screw v2 (Autodesk Fusion 360 design; units mm, degrees)
Autodesk Fusion 360 part; units mm, degrees
note: some values were not read from the file. Set by a fixed rule: which sketch regions a step uses.
sketch "Sketch1" plane through (0, 0, 0) normal (0, 0, 1) x (1, 0, 0)
  circle A0 centre (0, 0) radius 5.574
  dimension "d2" = 11.148
  constraint coincident A0.centre origin
  measures "d2" diameter of A0
extrude "Extrude1" add sketch "Sketch1" along normal blind 15
thread "Thread1" "ISO Metric Trapezoidal Threads 14.0 TR14x3 7e" major diameter 13.882 minor diameter 10.3175 pitch 3 angle 30 modelled right hand crest width 1.0769 on face at (5.5463, -0.555, 10) crest through (6.941, 0, -0.75)
sketch "Sketch2" plane through (0, 0, 15) normal (0, 0, 1) x (-1, 0, 0)
  line L0 (-10, 0) -> (-5, -8.6603)
  line L1 (-5, -8.6603) -> (5, -8.6603)
  line L2 (5, -8.6603) -> (10, 0)
  line L3 (10, 0) -> (5, 8.6603)
  line L4 (5, 8.6603) -> (-5, 8.6603)
  line L5 (-5, 8.6603) -> (-10, 0)
  spline S0 degree 3 poles (6.2708, -2.9757) (6.4311, -2.1502) (6.4357, -1.3016) (6.1375, 0.1707) (5.9003, 0.7954) (5.2456, 1.882) (4.8488, 2.3466) (4.3786, 2.7277) knots 0 0 0 0 0.252255 0.252255 0.451709 0.451709 0.634339 0.634339 0.634339 0.634339
  arc A0 (4.3786, 2.7277) -> (-4.3786, 2.7277) centre (0, 0) ccw
  spline S1 degree 3 poles (-4.3786, 2.7277) (-4.9039, 2.302) (-5.3371, 1.7726) (-5.9952, 0.5792) (-6.2131, -0.0769) (-6.4329, -1.4913) (-6.4131, -2.243) (-6.2708, -2.9757) knots 0 0 0 0 0.202813 0.202813 0.407757 0.407757 0.63033 0.63033 0.63033 0.63033
  arc A1 (-6.2708, -2.9757) -> (6.2708, -2.9757) centre (0, 0) ccw
  dimension "d5" = 10
  constraint coincident A0.centre A1.centre
  measures "d5" distance of L0.start A0.centre
extrude "Extrude2" add sketch "Sketch2" along normal blind 4 contours L0 L1 L2 L3 L4 L5 | S0 A0 S1 A1
